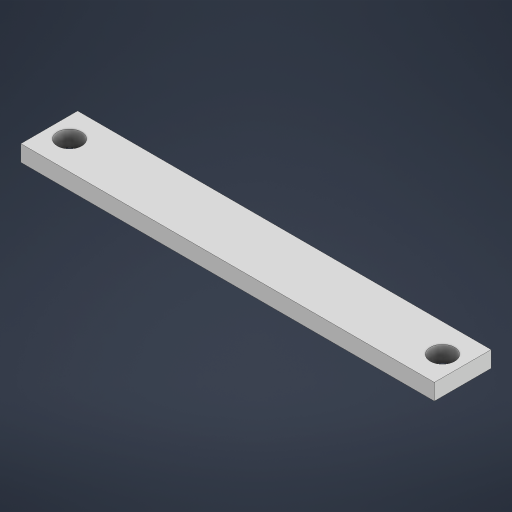
# Autodesk Inventor part: SAW_clamp_v2_top
Saved by Autodesk Inventor 2024.2 (Build 282272000, 272)
## iProperties
Created: 2024-04-15
Part Number: SAW_clamp_v2_top
Material: Generic
Document SubType Name: Modeling
Designer: magn1
Density: 1 g/cm^3
Appearance: Default
Author: magn1
Autodesk Inventor part; units mm, degrees
ref_plane "YZ Plane" through (0, 0, 0) normal (1, 0, 0) x (0, 1, 0)
ref_plane "XZ Plane" through (0, 0, 0) normal (0, 1, 0) x (-1, 0, 0)
ref_plane "XY Plane" through (0, 0, 0) normal (0, 0, 1) x (1, 0, 0)
sketch "Sketch1" plane through (0, 0, 0) normal (0, 0, 1) x (1, 0, 0)
  line L0 (17, -8.875) -> (-17, -8.875) construction
  line L1 (-17, -8.875) -> (-17, 8.875) construction
  line L2 (-17, 8.875) -> (17, 8.875) construction
  line L3 (17, 8.875) -> (17, -8.875) construction
  line L4 (17, -8.875) -> (-17, 8.875) construction
  line L5 (-17, -8.875) -> (17, 8.875) construction
  line L6 (20.5, 12.375) -> (-20.5, 12.375)
  line L7 (-20.5, 12.375) -> (-20.5, -12.375)
  line L8 (-20.5, -12.375) -> (20.5, -12.375)
  line L9 (20.5, -12.375) -> (20.5, 12.375)
  line L10 (20.5, 12.375) -> (-20.5, -12.375) construction
  line L11 (-20.5, 12.375) -> (20.5, -12.375) construction
  line L12 (-25.5, -14.375) -> (25.5, -14.375)
  line L13 (25.5, -14.375) -> (25.5, 14.375)
  line L14 (25.5, 14.375) -> (-25.5, 14.375)
  line L15 (-25.5, 14.375) -> (-25.5, -14.375)
  line L16 (-25.5, -14.375) -> (25.5, 14.375) construction
  line L17 (25.5, -14.375) -> (-25.5, 14.375) construction
  line L18 (-20.5, 12.375) -> (-25.5, 12.375)
  line L19 (20.5, 12.375) -> (25.5, 12.375)
  point P0 (0, 0)
  dimension "d0" = 34
  dimension "d1" = 17.75
  dimension "d2" = 41
  dimension "d3" = 24.75
  dimension "d4" = 51
  dimension "d5" = 28.75
  constraints: 40 end point, 6 midpoint, 6 parallel, 4 perpendicular, 3 horizontal, 3 point on line
  measures "d0" distance of L1.end L2.end
  measures "d1" distance of L0.end L1.end
  measures "d2" distance of L8.end L7.end
  measures "d3" distance of L7.end L6.end
  measures "d4" distance of L14.end L13.end
  measures "d5" distance of L13.end L12.end
extrude "Extrusion1" add sketch "Sketch1" along normal blind 7 contours L6 L18 L15 L14 L13 L19
sketch "Sketch3" plane through (-25.5, 14.375, 0) normal (0, 1, 0) x (1, 0, 0)
  line L0 (0, 0) -> (0, -7) construction
  line L1 (0, -3.5) -> (2.5, -3.5) construction
  line L2 (51, 0) -> (51, -7) construction
  line L3 (51, -3.5) -> (48.5, -3.5) construction
  line L4 (51, -3.5) -> (53.5, -3.5) construction
  circle A0 centre (2.5, -3.5) radius 1.5
  circle A1 centre (48.5, -3.5) radius 1.5
  point P0 (25.5, 0)
  dimension "d18" = 2.5
  dimension "d19" = 2.5
  dimension "d20" = 180
  dimension "d21" = 3
  dimension "d22" = 3
  constraints: 6 end point, 3 horizontal, 2 centre point, 2 coincident, 2 midpoint, 1 collinear
  measures "d18" distance of L1.start L1.end
  measures "d19" distance of L3.start L3.end
  measures "d20" angle of L3 L4
  measures "d21" diameter of A0
  measures "d22" diameter of A1
extrude "Extrusion3" cut sketch "Sketch3" against normal through all
body "Solid1"
